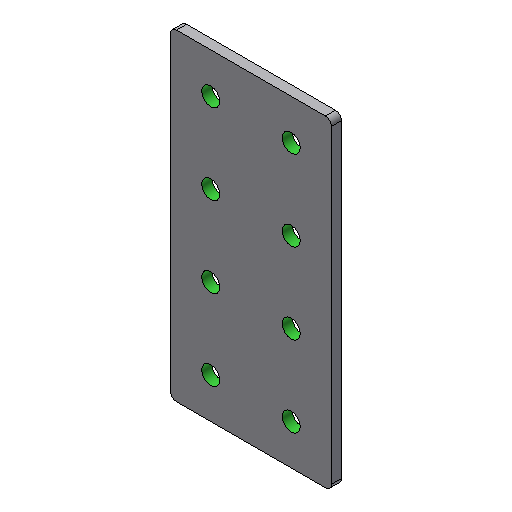
# Autodesk Inventor part: TL20240701-10130CV-004
Saved by Autodesk Inventor 2022.5 (Build 265521000, 521)
## iProperties
Category: JOINT LEG ASSY
Company: 현대 트랜시스(대유)
Created: 2023-04-20
Part Number: TL20240701-10130CV-004
Checked By: 김형민
Engr Approved By: 김시현
User Status: 2 x37
Material: SS400
Description: 0
Document SubType Name: Modeling
Mfg Approved By: 호상태
Designer: 김건휴
Stock Number: 004
Density: 7.85 g/cm^3
Appearance: Painting-RAL7035
Project: SW PJT
DETAIL: Coveryor Assembly
M/C TITLE: CJ 제일제당 협동로봇 포장시스탬 PILOT 장비
PARTS NAME: Bracket
SPECIFICATION: TA20221101-CV200000-015
DocNumber: 221118_Standard_v1
Folder: .\
VDS_Category: 엔지니어링
Detail Description: Processed products
Title: PLATE
Subject: SW차종 시트조립라인
Author: 김건휴
Revision Number: A
Autodesk Inventor part; units mm, degrees
ref_plane "YZ Plane" through (0, 0, 0) normal (1, 0, 0) x (0, 1, 0)
ref_plane "XZ Plane" through (0, 0, 0) normal (0, 1, 0) x (-1, 0, 0)
ref_plane "XY Plane" through (0, 0, 0) normal (0, 0, 1) x (1, 0, 0)
sketch "스케치9" plane through (0, 0, 0) normal (0, 0, 1) x (1, 0, 0)
  line L0 (-40, 80) -> (40, 80)
  line L1 (40, 80) -> (40, -80)
  line L2 (40, -80) -> (-40, -80)
  line L3 (-40, -80) -> (-40, 80)
  line L4 (-40, 80) -> (40, -80) construction
  line L5 (40, 80) -> (-40, -80) construction
  point P0 (0, 0)
  dimension "d40" = 80
  dimension "d41" = 160
  constraints: 12 end point, 2 midpoint, 2 parallel, 1 horizontal, 1 perpendicular
  measures "d40" distance of L0.start L0.end
  measures "d41" distance of L0.end L1.end
extrude "돌출4" add sketch "스케치9" along normal mid plane 5
sketch "스케치10" plane through (0, 0, 2.5) normal (0, 0, 1) x (1, 0, 0)
  line L0 (-20, 60) -> (20, 60)
  line L1 (20, 60) -> (20, 20)
  line L2 (20, 20) -> (-20, 20)
  line L3 (-20, 20) -> (-20, 60)
  line L4 (-20, 60) -> (20, 20) construction
  line L5 (20, 60) -> (-20, 20) construction
  line L6 (-20, -20) -> (20, -20)
  line L7 (20, -20) -> (20, -60)
  line L8 (20, -60) -> (-20, -60)
  line L9 (-20, -60) -> (-20, -20)
  line L10 (-20, -20) -> (20, -60) construction
  line L11 (20, -20) -> (-20, -60) construction
  line L12 (40, 80) -> (-40, 80) projected
  point P0 (0, 0)
  point P1 (0, 40)
  point P2 (0, -40)
  point P3 (0, 40)
  point P4 (0, -40)
  dimension "d44" = 40
  dimension "d45" = 40
  dimension "d46" = 40
  dimension "d47" = 40
  dimension "d48" = 40
  dimension "d49" = 20
  dimension "d50" = 20
  constraints: 24 end point, 6 midpoint, 4 parallel, 2 horizontal, 2 perpendicular, 1 vertical alignment
  measures "d44" distance of L0.start L0.end
  measures "d45" distance of L2.end L0.start
  measures "d46" distance of L8.end L6.start
  measures "d47" distance of L6.start L6.end
  measures "d48" distance between parallel lines of L6 L2
  measures "d49" horizontal distance of L0.start L12.end
  measures "d50" distance between parallel lines of L12 L0
hole "구멍3" at (20, 60, 2.5) at (-20, 60, 2.5) at (20, 20, 2.5) at (-20, 20, 2.5) at (20, -20, 2.5) at (-20, -20, 2.5) at (20, -60, 2.5) at (-20, -60, 2.5) direction (0, 0, -1) diameter 9 end through all clearance for "Socket Head Cap Screw ISO 4762" size "M8" standard "ISO"
fillet "모깎기2" radius 3 4 edges at (40, 80, 0) (-40, 80, 0) (40, -80, 0) (-40, -80, 0)
